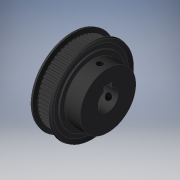
# Autodesk Inventor part: GPA60GT2060-B-NK10_b
Saved by Autodesk Inventor 2019 (Build 230136000, 136)
## iProperties
Created: 2022-10-05
Part Number: GPA60GT2060-B-NK10_b
Material: Generic
Catalog Web Link: www.cadenas.de
Description: GPA_GT2040, GPA_GT2060, GPA_GT2090, KGPA_GT2040, KGPA_GT2060, KGPA_GT2090, KGPK_GT2040, KGPK_GT2060, KGPK_GT2090_body-High Torque Timing Pulleys 2GT Type
Vendor: MISUMI
Document SubType Name: Modeling
Designer: psAdmin
Manufacturer: MISUMI
Mass: 14.3886 g
Surface Area: 62.1682 cm^2
Volume: 14.3886 cm^3
Density: 1 g/cm^3
Appearance: PSOLRGB-175-175-175
Category: PARTsolutions
Company: MISUMI
Title: GPA60GT2060-B-NK10
Author: Cadenas PARTsolutions
Comments: High Torque Timing Pulleys 2GT Type
PSOL_IDENT_0: {$CADENAS_DATA/23d-libs/misumi/metric/51_timing_pulleys/gpa__gt2/gpa_gt2.prj},481 {VTYP=3D},{NB=GPA6
PSOL_IDENT_1: 0GT2060-B-NK10_b},{LINA=GPA60GT2060-B-NK10},{NN=GPA_GT2040, GPA_GT2060, GPA_GT2090, KGPA_GT2040, KGP
PSOL_IDENT_2: A_GT2060, KGPA_GT2090, KGPK_GT2040, KGPK_GT2060, KGPK_GT2090_body},{DATE=25.04.2022 01:22:58},{GEOMD
PSOL_IDENT_3: ATE=22.12.2021 00:45:33},{VERSION=},{LINEID=190},{WBVAR=MAT,ST,TNW,PS,SBS,DD,Z,J,Q,R,S,T,ALT1,ALT2,M
PSOL_IDENT_4: ,QSC,QFC,QTC,ALT3,K,KSC,KFC,KTC,ALT4,ZM,ZSC,ZFC,ZTC,ALT5,BC,ALT6,ALT7,ALT8,FC,ALT13,BN},{WBNUMERIC=D
PSOL_IDENT_5: D,Z,J,Q,R,S,T,QSC,QFC,QTC,K,KSC,KFC,KTC,ZSC,ZFC,ZTC,BC,FC,BN}  {NB=GPA60GT2060-B-NK10_b},{LINA=GPA60
PSOL_IDENT_6: GT2060-B-NK10},{KT=DUMMY},{PN=GPA60GT2060-B-NK10},{TYPE=GPA},{MAT=AA},{ST=CA},{NT=60},{TNW=GT2060},{
PSOL_IDENT_7: BW=6},{A=7.0},{W=10.3},{L=18.0},{PS=B},{PSA= 'A','B' },{SBS=NK},{SBSALG= 'H','Round Hole','P','Round
PSOL_IDENT_8: Hole+Tap','N','New JIS Keywayed Bore + Tap (Standard)','NK','New JIS Keywayed Bore + Tap (keyway wi
PSOL_IDENT_9: dth 4.0mm, height 1.8mm)','V','Stepped Hole','F','Stepped Hole (Counterbore holes on the boss side)'
PSOL_IDENT_10: },{DD=10.00},{DDALG=[10:10/1]},{DDHA=[8:29/1]},{DDHB=[8:24/1]},{DDPA=[8:22/1]},{DDPB=[8:22/1]},{DDN
PSOL_IDENT_11: A=8,10,11,12,13,14,15,16,17,18,19},{DDNB=8,10,11,12,13,14},{DDNKA=[10:10/1]},{DDNKB=[10:10/1]},{DDVA=
PSOL_IDENT_12: [8:27/1]},{DDVFB=[8:22/1]},{DDYA=[8:27/1]},{Z=0},{ZALG=0},{ZMIN=12},{ZAMAX=29},{ZBMAX=24},{J=0.0},{J
PSOL_IDENT_13: ALG=0},{JMAX=16},{Q=0},{R=0},{QRALG=0},{QRMIN=12},{QRMAX=29},{S=0.0},{SALG=0},{SMAX=4.300},{T=0.0},{
PSOL_IDENT_14: TALG=0},{TMAX=5.000},{PD=38.20},{OD=37.69},{D=28},{DE=28},{DDZ=10},{F=42},{E=33},{BB=4},{TT=1.8},{M1=
PSOL_IDENT_15: 4},{AC=M4x3},{ALT1=},{ALT1A= '','w/o Set Screw Angle','-KC90','with KC90 (Set Screw Angle)' },{ANG=1
PSOL_IDENT_16: 20},{ALT2=},{ALT2A= '','w/o Side Tapped Hole','-QTC','with QTC (3 Places Side Tapped Hole)' },{M=N/A
PSOL_IDENT_17: },{MALG= 'N/A' },{MM=0.000},{MPHD=0.000},{MA= 'N/A' },{MSA= 'N/A' },{QSC=0.0},{QSCA=0},{QFC=0.0},{QF
PSOL_IDENT_18: CA=0},{QTC=0.0},{QTCA=0},{QPCDMIN=14},{QPCDMINALG=14},{QPCDMAX=24},{ALT2PN=},{ALT3=},{ALT3A= '','w/o
PSOL_IDENT_19: Side Through Hole','-KTC','with KTC (3 Places Side Through Hole)' },{K=0.0},{KA=0},{KAMIN=4},{KAMAX=
PSOL_IDENT_20: 5},{KSMAX=5},{KSC=0.0},{KSCA=0},{KFC=0.0},{KFCA=0},{KTC=0.0},{KTCA=0},{KSCMIN=14.000},{KPCDMIN=14.00
PSOL_IDENT_21: 0},{KPCDMINALG=18.000},{KPCDMAX=24.000},{ALT3PN=},{ALT4=},{ALT4ALG= '','w/o Side Counterbored','ZTC'
PSOL_IDENT_22: ,'with ZTC (3 Places Side Counterbored)' },{ALT4MIN=20.500},{ALT4MAX=20.500},{ZM=N/A},{ZMALG= 'N/A'
PSOL_IDENT_23: },{ZMFTALG= 'N/A' },{ZMSALG= 'N/A' },{ZMDD1=0.0},{ZMDD2=0.0},{ZMHH=0.0},{ZSC=0.0},{ZSCALG=[0]},{ZFC=
PSOL_IDENT_24: 0.0},{ZFCALG=[0]},{ZTC=0.0},{ZTCALG=[0]},{ZPCDMIN=0.000},{ZPCDMINALG=0.000},{ZPCDMAX=24.000},{ALT4PN=
PSOL_IDENT_25: },{ALT5=},{ALT5ALG= '','w/o BC (Boss Cut)','-BC','with BC (Boss Cut)' },{ALT5PN=},{BC=0.0},{BCALG=0}
PSOL_IDENT_26: ,{BCMIN=7.000},{BCMAX=7.700},{ALT6=},{ALT7=},{ALT7ALG= '','w/o Flange Attached on One Side Only','-R
PSOL_IDENT_27: FC','with RFC (Flange Attached on The Boss Side Only)','-LFC','with LFC (Flange Attached on The Oppo
PSOL_IDENT_28: site Side Only)' },{ALT8=},{ALT8ALG='','w/o FC (Flange Cut)','-FC','with FC (Flange Cut)'},{ALT8PN=}
PSOL_IDENT_29: ,{FC=0.0},{FCA=0},{ODAINT=41.000},{FCMIN=39},{FCMAX=40},{WLBC=18},{SL=6.8},{SL2=5},{KTT=5},{KYY=7.2}
PSOL_IDENT_30: ,{TAP=0},{MATALG= 'AA','Aluminum Alloy 2000 series' , '6000','6000 Series Aluminum Alloy' },{STALG= '
PSOL_IDENT_31: CA','Clear Anodize' },{ALT13=},{BN=0.000},{BNMIN=8.200},{BNMAX=17.700},{ALT13ALG= '','w/o BN (Hub Le
PSOL_IDENT_32: ngthening)','BN','with BN (Hub Lengthening)' },{BNALG=0},{BNPN=}
NB: GPA60GT2060-B-NK10_b
NN: GPA_GT2040, GPA_GT2060, GPA_GT2090, KGPA_GT2040, KGPA_GT2060, KGPA_GT2090, KGPK_GT2040, KGPK_GT2060, KGPK_GT2090_body
NT: 60
NBSYN: $PN._b
LINA: GPA60GT2060-B-NK10
CATALOG: Misumi
PN: GPA60GT2060-B-NK10
MAT: Aluminum Alloy 2000 series
ST: Clear Anodize
TNW: GT2060
A: 7
W: 10.3
L: 18
PS: B
SBS: New JIS Keywayed Bore + Tap (keyway width 4.0mm, height 1.8mm)
DD: 10
Z: 0
J: 0
Q: 0
R: 0
S: 0
T: 0
PD: 38.2
OD: 37.69
D: 28
F: 42
E: 33
AC: M4x3
ALT1: w/o Set Screw Angle
ALT2: w/o Side Tapped Hole
M: N/A
QSC: 0
QFC: 0
QTC: 0
ALT3: w/o Side Through Hole
K: 0
KSC: 0
KFC: 0
KTC: 0
ALT4: w/o Side Counterbored
ZM: N/A
ZMDD1: 0
ZMDD2: 0
ZMHH: 0
ZSC: 0
ZFC: 0
ZTC: 0
ALT5: w/o BC (Boss Cut)
BC: 0
ALT6: w/o Flange not Attached
ALT7: w/o Flange Attached on One Side Only
ALT8: w/o FC (Flange Cut)
FC: 0
ALT13: w/o BN (Hub Lengthening)
BN: 0
SUPPLIER: MISUMI
ARTICLENO: GPA60GT2060-B-NK10_b
BOMINFO: GPA60GT2060-B-NK10
CREATOR: CADENAS GmbH
Autodesk Inventor part; units mm, degrees
ref_plane "YZ Plane" through (0, 0, 0) normal (1, 0, 0) x (0, 1, 0)
ref_plane "XZ Plane" through (0, 0, 0) normal (0, 1, 0) x (-1, 0, 0)
ref_plane "XY Plane" through (0, 0, 0) normal (0, 0, 1) x (1, 0, 0)
sketch "Sketch_17" plane through (0, 0, 0) normal (0, 0, 1) x (1, 0, 0)
  line L0 (12.85, 0) -> (-5.15, 0)
  line L1 (-5.15, 0) -> (-5.15, 16.5)
  line L2 (-5.15, 16.5) -> (-3.5, 16.5)
  line L3 (-3.5, 16.5) -> (-3.5, 18.845)
  line L4 (-3.5, 18.845) -> (3.5, 18.845)
  line L5 (3.5, 18.845) -> (3.5, 16.5)
  line L6 (3.5, 16.5) -> (5.15, 16.5)
  line L7 (5.15, 16.5) -> (5.15, 14)
  line L8 (5.15, 14) -> (12.85, 14)
  line L9 (12.85, 14) -> (12.85, 0)
  line L10 (12.85, 0) -> (-5.15, 0)
  constraints: 22 end point
revolve "Revolution1" add sketch "Sketch_17" angle 360 about axis through (12.85, 0, 0) along (1, 0, 0)
sketch "Sketch_18" plane through (0, 0, 0) normal (1, 0, 0) x (0, 1, 0)
  line L0 (19.0763, 0.9521) -> (18.8232, 0.9394)
  line L1 (18.8232, 0.9394) -> (18.8294, 0.7899)
  arc A0 (18.7251, 0.6734) -> (18.8294, 0.7899) centre (18.7175, 0.7852) ccw
  arc A1 (18.7251, 0.6734) -> (18.7251, -0.6734) centre (18.771, 0) ccw
  arc A2 (18.8294, -0.7899) -> (18.7251, -0.6734) centre (18.7175, -0.7852) ccw
  line L2 (18.8294, -0.7899) -> (18.8232, -0.9394)
  line L3 (18.8232, -0.9394) -> (19.0763, -0.9521)
  arc A3 (19.0763, -0.9521) -> (19.0763, 0.9521) centre (0, 0) ccw
  constraints: 8 end point, 8 point on circle, 4 centre point
extrude "Extrusion1" cut sketch "Sketch_18" along normal mid plane 7
pattern_circular "Circular Pattern1" count 60 over 360 about axis through (0, 0, 0) along (1, 0, 0) of "Extrusion1"
sketch "Sketch_20" plane through (0, 0, 0) normal (0, 0, 1) x (1, 0, 0)
  line L0 (50, 0) -> (-50, 0)
  line L1 (3.5, 18.845) -> (3.5, 16.5)
  line L2 (3.5, 16.5) -> (4.5, 16.5)
  line L3 (4.5, 16.5) -> (4.5, 18.7133)
  line L4 (4.5, 18.7133) -> (5.0434, 20.7412)
  line L5 (5.0434, 20.7412) -> (4.0774, 21)
  line L6 (4.0774, 21) -> (3.5, 18.845)
  constraints: 14 end point
revolve "Revolution2" add sketch "Sketch_20" angle 360 about axis through (50, 0, 0) along (1, 0, 0)
sketch "Sketch_21" plane through (0, 0, 0) normal (0, 0, 1) x (1, 0, 0)
  line L0 (50, 0) -> (-50, 0)
  line L1 (-5.0434, 20.7412) -> (-4.5, 18.7133)
  line L2 (-4.5, 18.7133) -> (-4.5, 16.5)
  line L3 (-4.5, 16.5) -> (-3.5, 16.5)
  line L4 (-3.5, 16.5) -> (-3.5, 18.845)
  line L5 (-3.5, 18.845) -> (-4.0774, 21)
  line L6 (-4.0774, 21) -> (-5.0434, 20.7412)
  constraints: 14 end point
revolve "Revolution3" add sketch "Sketch_21" angle 360 about axis through (50, 0, 0) along (1, 0, 0)
sketch "Sketch_1" plane through (8.85, 0, 0) normal (1, 0, 0) x (0, 0, -1)
  line L0 (0, 0) -> (0, 14)
  line L1 (0, 14) -> (1.621, 14)
  line L2 (1.621, 14) -> (1.621, 0)
  line L3 (1.621, 0) -> (0, 0)
  line L4 (0, 0) -> (0, 14)
  constraints: 10 end point
revolve "Revolution4" cut sketch "Sketch_1" angle 360 about axis through (8.85, 0, 0) along (0, -1, 0)
thread "Thread1" size "M4x0.7" class "6H" standard "ISO Metric profile" length 7.2
sketch "Sketch_2" plane through (8.85, 0, 0) normal (1, 0, 0) x (0, 0, -1)
  line L0 (0, 0) -> (12.1244, -7)
  line L1 (12.1244, -7) -> (11.3139, -8.4038)
  line L2 (11.3139, -8.4038) -> (-0.8105, -1.4038)
  line L3 (-0.8105, -1.4038) -> (0, 0)
  line L4 (0, 0) -> (12.1244, -7)
  constraints: 10 end point
revolve "Revolution5" cut sketch "Sketch_2" angle 360 about axis through (8.85, 0, 0) along (0, 0.5, 0.8660254)
thread "Thread2" size "M4x0.7" class "6H" standard "ISO Metric profile" length 9
sketch "Sketch_3" plane through (-5.15, 0, 0) normal (1, 0, 0) x (0, 0, -1)
  arc A0 (-2, 4.5826) -> (2, 4.5826) centre (0, 0) ccw
  line L0 (2, 4.5826) -> (2, 6.8)
  line L1 (2, 6.8) -> (-2, 6.8)
  line L2 (-2, 6.8) -> (-2, 4.5826)
  constraints: 6 end point, 2 point on circle, 1 centre point
extrude "Extrusion2" cut sketch "Sketch_3" along normal blind 18
ref_plane "to_screw_B1_XY" through (8.85, 6.8, 0) normal (0, 1, 0) x (1, 0, 0)
ref_plane "to_screw_B1_YZ" through (8.85, 6.8, 0) normal (1, 0, 0) x (0, 0, -1)
ref_plane "to_screw_B1_ZX" through (8.85, 6.8, 0) normal (0, 0, -1) x (0, 1, 0)
ref_plane "to_screw_B2_XY" through (8.85, -2.5, -4.3301) normal (0, -0.5, -0.8660254) x (1, 0, 0)
ref_plane "to_screw_B2_YZ" through (8.85, -2.5, -4.3301) normal (1, 0, 0) x (0, -0.8660254, 0.5)
ref_plane "to_screw_B2_ZX" through (8.85, -2.5, -4.3301) normal (0, -0.8660254, 0.5) x (0, -0.5, -0.8660254)
body "Solid1"
